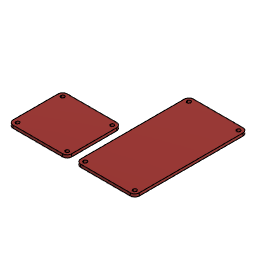
Lower Bay Tray - Template (Autodesk Fusion 360 design; units mm, degrees)
Autodesk Fusion 360 part; units mm, degrees
sketch "Sketch1" plane through (0, 0, 0) normal (0, 0, 1) x (1, 0, 0)
  line L0 (-65, 70) -> (-10, 70) construction
  line L1 (-10, 70) -> (-10, 20) construction
  line L2 (-10, 20) -> (-65, 20) construction
  line L3 (-65, 20) -> (-65, 70) construction
  line L4 (-70, 20) -> (-70, 70)
  arc A0 (-65, 75) -> (-70, 70) centre (-65, 70) ccw
  arc A1 (-5, 70) -> (-10, 75) centre (-10, 70) ccw
  line L5 (-5, 70) -> (-5, 20)
  line L6 (-65, 75) -> (-10, 75)
  arc A2 (-70, 20) -> (-65, 15) centre (-65, 20) ccw
  line L7 (-10, 15) -> (-65, 15)
  arc A3 (-10, 15) -> (-5, 20) centre (-10, 20) ccw
  line L8 (-66.8, 70.25) -> (-66.8, 69.75)
  arc A4 (-66.8, 69.75) -> (-63.2, 69.75) centre (-65, 69.75) ccw
  line L9 (-63.2, 69.75) -> (-63.2, 70.25)
  arc A5 (-63.2, 70.25) -> (-66.8, 70.25) centre (-65, 70.25) ccw
  line L10 (-65, 70.25) -> (-65, 69.75) construction
  line L11 (-37.5, 75) -> (-37.5, 15) construction
  line L12 (-70, 45) -> (-5, 45) construction
  arc A6 (-66.8, 19.75) -> (-63.2, 19.75) centre (-65, 19.75) ccw
  line L13 (-66.8, 19.75) -> (-66.8, 20.25)
  arc A7 (-63.2, 20.25) -> (-66.8, 20.25) centre (-65, 20.25) ccw
  line L14 (-63.2, 20.25) -> (-63.2, 19.75)
  arc A8 (-8.2, 70.25) -> (-11.8, 70.25) centre (-10, 70.25) ccw
  line L15 (-8.2, 70.25) -> (-8.2, 69.75)
  arc A9 (-11.8, 69.75) -> (-8.2, 69.75) centre (-10, 69.75) ccw
  line L16 (-11.8, 69.75) -> (-11.8, 70.25)
  line L17 (-11.8, 20.25) -> (-11.8, 19.75)
  arc A10 (-8.2, 20.25) -> (-11.8, 20.25) centre (-10, 20.25) ccw
  line L18 (-8.2, 19.75) -> (-8.2, 20.25)
  arc A11 (-11.8, 19.75) -> (-8.2, 19.75) centre (-10, 19.75) ccw
  line L19 (70, 140) -> (70, 15) construction
  line L20 (70, 15) -> (5, 15) construction
  line L21 (5, 140) -> (70, 140) construction
  line L22 (5, 15) -> (5, 140) construction
  line L23 (10, 135) -> (65, 135) construction
  line L24 (65, 135) -> (65, 20) construction
  line L25 (65, 20) -> (10, 20) construction
  line L26 (10, 20) -> (10, 135) construction
  line L27 (65, 15) -> (10, 15)
  line L28 (5, 20) -> (5, 135)
  line L29 (10, 140) -> (65, 140)
  line L30 (70, 135) -> (70, 20)
  arc A12 (10, 140) -> (5, 135) centre (10, 135) ccw
  arc A13 (70, 135) -> (65, 140) centre (65, 135) ccw
  arc A14 (5, 20) -> (10, 15) centre (10, 20) ccw
  arc A15 (65, 15) -> (70, 20) centre (65, 20) ccw
  line L31 (8.1, 135.25) -> (8.1, 134.75)
  arc A16 (8.1, 134.75) -> (11.9, 134.75) centre (10, 134.75) ccw
  line L32 (11.9, 134.75) -> (11.9, 135.25)
  arc A17 (11.9, 135.25) -> (8.1, 135.25) centre (10, 135.25) ccw
  line L33 (10, 135.25) -> (10, 134.75) construction
  line L34 (37.5, 140) -> (37.5, 15) construction
  line L35 (5, 77.5) -> (70, 77.5) construction
  arc A18 (63.1, 134.75) -> (66.9, 134.75) centre (65, 134.75) ccw
  line L36 (63.1, 134.75) -> (63.1, 135.25)
  arc A19 (66.9, 135.25) -> (63.1, 135.25) centre (65, 135.25) ccw
  line L37 (66.9, 135.25) -> (66.9, 134.75)
  line L38 (66.9, 19.75) -> (66.9, 20.25)
  arc A20 (63.1, 19.75) -> (66.9, 19.75) centre (65, 19.75) ccw
  line L39 (63.1, 20.25) -> (63.1, 19.75)
  arc A21 (66.9, 20.25) -> (63.1, 20.25) centre (65, 20.25) ccw
  arc A22 (8.1, 19.75) -> (11.9, 19.75) centre (10, 19.75) ccw
  line L40 (8.1, 19.75) -> (8.1, 20.25)
  line L41 (11.9, 20.25) -> (11.9, 19.75)
  arc A23 (11.9, 20.25) -> (8.1, 20.25) centre (10, 20.25) ccw
  line L42 (-10, 15) -> (5, 15) construction
  line L43 (0, 0) -> (0, 15) construction
  point P0 (-65, 70)
  point P1 (10, 135)
  point P2 (65, 135)
  point P3 (10, 20)
  point P4 (65, 20)
  point P5 (10, 135)
  dimension "d1" = 3.6
  dimension "d5" = 3.8
  dimension "d25" = 65
  dimension "d26" = 125
  dimension "d27" = 60
  dimension "d28" = 65
  dimension "d29" = 55
  dimension "d30" = 55
  dimension "d31" = 115
  dimension "d32" = 50
  dimension "d33" = 5
  dimension "d34" = 5
  dimension "d35" = 5
  dimension "d36" = 5
  dimension "d37" = 5
  dimension "d38" = 5
  dimension "d39" = 5
  dimension "d40" = 5
  dimension "d41" = 5
  dimension "d42" = 15
  constraint tangent L8 A4
  constraint tangent A4 L9
  constraint parallel L8 L9
  constraint tangent L9 A5
  constraint tangent L8 A5
  constraint vertical L10
  constraint coincident P0 L0.start
  constraint midpoint L10 P0
  constraint midpoint L6 L11.start
  constraint midpoint L7 L11.end
  constraint midpoint L4 L12.start
  constraint midpoint L5 L12.end
  constraint symmetric L8.start L12 A6.start
  constraint symmetric L8.end L12 L13.end
  constraint symmetric A4.end L12 A7.start
  constraint symmetric L9.end L12 A6.end
  constraint symmetric A4 L12 A7
  constraint symmetric A5 L12 A6
  constraint symmetric L8.start L11 A8.start
  constraint symmetric L8.end L11 L15.end
  constraint symmetric A4.end L11 A9.start
  constraint symmetric L9.end L11 A8.end
  constraint symmetric A4 L11 A9
  constraint symmetric A5 L11 A8
  constraint symmetric L11 A6.end L17.end
  constraint symmetric L11 A6.start L18.start
  constraint symmetric L11 A6 A11
  constraint symmetric L11 L13.end A10.start
  constraint symmetric L11 A7.start L17.start
  constraint symmetric L11 A7 A10
  constraint horizontal L23
  constraint vertical L24
  constraint horizontal L25
  constraint vertical L26
  constraint coincident P4 L24.end
  constraint coincident P5 P1
  constraint coincident L21 L29.start
  constraint parallel L25 L27
  constraint parallel L26 L28
  constraint parallel L23 L29
  constraint parallel L24 L30
  constraint coincident L21 L29.end
  constraint coincident P2 L23.end
  constraint coincident L22 L28.start
  constraint coincident P3 L25.end
  constraint tangent L31 A16
  constraint tangent A16 L32
  constraint parallel L31 L32
  constraint tangent L32 A17
  constraint tangent L31 A17
  constraint vertical L33
  constraint midpoint L33 P5
  constraint midpoint L21 L34.start
  constraint midpoint L20 L34.end
  constraint midpoint L28 L35.start
  constraint midpoint L19 L35.end
  constraint symmetric L31.start L34 A19.start
  constraint symmetric L31.end L34 A18.end
  constraint symmetric A16.end L34 A18.start
  constraint symmetric L32.end L34 L36.end
  constraint symmetric A16 L34 A18
  constraint symmetric A17 L34 A19
  constraint symmetric L31.start L35 A22.start
  constraint symmetric L31.end L35 L40.end
  constraint symmetric A16.end L35 L41.start
  constraint symmetric L32.end L35 A22.end
  constraint symmetric A16 L35 A23
  constraint symmetric A17 L35 A22
  constraint symmetric L35 A18.end L38.end
  constraint symmetric L35 A18.start L39.start
  constraint symmetric L35 A18 A21
  constraint symmetric L35 L36.end A20.start
  constraint symmetric L35 A19.start L38.start
  constraint symmetric L35 A19 A20
  constraint tangent A3 L42
  constraint coincident L43.start origin
  constraint coincident L42 L43.end
  constraint perpendicular L42 L43
  constraint coincident L20 L22.start
  constraint coincident L20 L27.end
  constraint coincident L20 L27.start
  constraint coincident L7.start L42
  constraint coincident A2.end L7
  constraint coincident L4 A2.start
  measures "d1" diameter of A4
  measures "d5" diameter of A16
  measures "d25" distance of L22 L30
  measures "d26" distance of L21 L27
  measures "d27" distance of L6 L7
  measures "d28" distance of L4 L5
  measures "d29" distance of L1 L3
  measures "d30" distance of L24 L26
  measures "d31" distance of L23 L25
  measures "d32" distance of L0 L2
  measures "d33" radius of A2
  measures "d34" radius of A3
  measures "d35" radius of A1
  measures "d36" radius of A0
  measures "d37" radius of A15
  measures "d38" horizontal distance of L20.end P3
  measures "d39" radius of A13
  measures "d40" radius of A12
  measures "d41" distance of L5 L43
  measures "d42" distance of L7 L43.start
extrude "Extrude1" add sketch "Sketch1" along normal blind 3 contours L4 A0 A1 L5 L6 A2 L7 A3 makes body 1 in component "Small Template"
extrude "Extrude1'" add sketch "Sketch1" along normal blind 3 separate body contours L27 L28 L29 L30 A12 A13 A14 A15 makes body 2 in component "Large Template"
ref_plane "WorkPlane1" through (0, 0, 3) normal (0, 0, 1) x (1, 0, 0)
sketch "Sketch2" plane through (0, 0, 0) normal (0, 0, -1) x (1, 0, 0)
  arc A0 (63.1, -20.25) -> (66.9, -20.25) centre (65, -20.25) ccw
  line L0 (63.1, -20.25) -> (63.1, -19.75)
  arc A1 (66.9, -19.75) -> (63.1, -19.75) centre (65, -19.75) ccw
  line L1 (66.9, -19.75) -> (66.9, -20.25)
  arc A2 (8.1, -135.25) -> (11.9, -135.25) centre (10, -135.25) ccw
  line L2 (8.1, -135.25) -> (8.1, -134.75)
  arc A3 (11.9, -134.75) -> (8.1, -134.75) centre (10, -134.75) ccw
  line L3 (11.9, -134.75) -> (11.9, -135.25)
  arc A4 (11.9, -19.75) -> (8.1, -19.75) centre (10, -19.75) ccw
  line L4 (11.9, -19.75) -> (11.9, -20.25)
  arc A5 (8.1, -20.25) -> (11.9, -20.25) centre (10, -20.25) ccw
  line L5 (8.1, -20.25) -> (8.1, -19.75)
  arc A6 (66.9, -134.75) -> (63.1, -134.75) centre (65, -134.75) ccw
  line L6 (66.9, -134.75) -> (66.9, -135.25)
  arc A7 (63.1, -135.25) -> (66.9, -135.25) centre (65, -135.25) ccw
  line L7 (63.1, -135.25) -> (63.1, -134.75)
  arc A8 (10, -15) -> (5, -20) centre (10, -20) ccw
  line L8 (5, -20) -> (5, -135)
  arc A9 (5, -135) -> (10, -140) centre (10, -135) ccw
  line L9 (10, -140) -> (65, -140)
  arc A10 (65, -140) -> (70, -135) centre (65, -135) ccw
  line L10 (70, -135) -> (70, -20)
  arc A11 (70, -20) -> (65, -15) centre (65, -20) ccw
  line L11 (65, -15) -> (10, -15)
  arc A12 (-63.2, -19.75) -> (-66.8, -19.75) centre (-65, -19.75) ccw
  line L12 (-63.2, -19.75) -> (-63.2, -20.25)
  arc A13 (-66.8, -20.25) -> (-63.2, -20.25) centre (-65, -20.25) ccw
  line L13 (-66.8, -20.25) -> (-66.8, -19.75)
  arc A14 (-11.8, -70.25) -> (-8.2, -70.25) centre (-10, -70.25) ccw
  line L14 (-11.8, -70.25) -> (-11.8, -69.75)
  arc A15 (-8.2, -69.75) -> (-11.8, -69.75) centre (-10, -69.75) ccw
  line L15 (-8.2, -69.75) -> (-8.2, -70.25)
  arc A16 (-66.8, -70.25) -> (-63.2, -70.25) centre (-65, -70.25) ccw
  line L16 (-66.8, -70.25) -> (-66.8, -69.75)
  arc A17 (-63.2, -69.75) -> (-66.8, -69.75) centre (-65, -69.75) ccw
  line L17 (-63.2, -69.75) -> (-63.2, -70.25)
  arc A18 (-8.2, -19.75) -> (-11.8, -19.75) centre (-10, -19.75) ccw
  line L18 (-8.2, -19.75) -> (-8.2, -20.25)
  arc A19 (-11.8, -20.25) -> (-8.2, -20.25) centre (-10, -20.25) ccw
  line L19 (-11.8, -20.25) -> (-11.8, -19.75)
  arc A20 (-65, -15) -> (-70, -20) centre (-65, -20) ccw
  line L20 (-70, -20) -> (-70, -70)
  arc A21 (-70, -70) -> (-65, -75) centre (-65, -70) ccw
  line L21 (-65, -75) -> (-10, -75)
  arc A22 (-10, -75) -> (-5, -70) centre (-10, -70) ccw
  line L22 (-5, -70) -> (-5, -20)
  arc A23 (-5, -20) -> (-10, -15) centre (-10, -20) ccw
  line L23 (-10, -15) -> (-65, -15)
  line L24 (-65, -70) -> (-10, -70) construction
  line L25 (10, -134.75) -> (10, -135.25)
  line L26 (10, -135.25) -> (10, -135)
  line L27 (65, -135.25) -> (65, -134.75)
  line L28 (10, -135) -> (65, -135) construction
  dimension "d15" = 6
  dimension "d16" = 6
  text T0 "V1" font "Arial" height 6 align centre spacing 1 along the path L24 letters at x, y, angle (-42.6262, -62.412, 0) (-37.0355, -62.412, 0)
  text T1 "v1" font "Arial" height 6 align centre spacing 1 along the path L28 letters at x, y, angle (33.0737, -127.412, 0) (37.2647, -127.412, 0)
  constraint coincident A21.centre L24.start
  constraint coincident A22.centre L24.end
  constraint coincident A3.centre L25.start
  constraint coincident A2.centre L25.end
  constraint coincident A9.centre L26.end
  constraint horizontal L28
  constraint coincident A7.centre L27.start
  constraint coincident A6.centre L27.end
extrude "Extrude3" cut sketch "Sketch2" against normal blind 0.4 text T0 bodies 1 in component "Small Template"
extrude "Extrude3'" cut sketch "Sketch2" against normal blind 0.4 text T1 bodies 2 in component "Large Template"
component "Small Template" placed x (1, 0, 0) y (0, 1, 0) z (0, 0, 1) at (0, 0, 0)
component "Large Template" placed x (1, 0, 0) y (0, 1, 0) z (0, 0, 1) at (0, 0, 0)
equation "large_m4 = 4.6 mm"
equation "small_m4 = 3.8 mm"
equation "large_m3 = 3.6 mm"
equation "small_m3 = 2.8 mm"
equation "d34 = d33"
equation "d35 = d33"
equation "d36 = d33"
equation "d37 = d33"
equation "d38 = d33"
equation "d39 = d33"
equation "d40 = d33"
